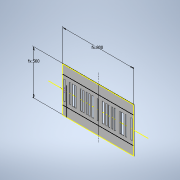
# Autodesk Inventor part: ferrite_layer_dex_1R1
Saved by Autodesk Inventor 2021 (Build 250183000, 183)
## iProperties
Created: 2021-01-27
Part Number: ferrite_layer_dex_1R1
Material: Generic
Document SubType Name: Modeling
Designer: pduy110
Density: 1 g/cm^3
Appearance: Default
Author: pduy110
Autodesk Inventor part; units mm, degrees
ref_plane "YZ Plane" through (0, 0, 0) normal (1, 0, 0) x (0, 1, 0)
ref_plane "XZ Plane" through (0, 0, 0) normal (0, 1, 0) x (-1, 0, 0)
ref_plane "XY Plane" through (0, 0, 0) normal (0, 0, 1) x (1, 0, 0)
sketch "ferrite_layer_outline_sketch" plane through (0, 0, 0) normal (0, 0, 1) x (1, 0, 0)
  line L0 (0, 250) -> (800, 250)
  line L1 (800, 250) -> (800, -250)
  line L2 (800, -250) -> (0, -250)
  line L3 (0, -250) -> (0, 250)
  line L4 (-160, 0) -> (960, 0) projected
  line L5 (400, 250) -> (400, -250) construction
  line L6 (400, 366.8869) -> (400, -324.3455) construction
  line L7 (400, 250) -> (400, -250)
  point P0 (0, 0)
  point P1 (0, 0)
  point P2 (0, 0)
  point P3 (0, 0)
  point P4 (20, 0)
  dimension "d0" = 800
  dimension "d1" = 500
  constraints: 14 end point, 3 coincident, 3 midpoint, 3 point on line, 2 parallel, 1 collinear, 1 horizontal, 1 perpendicular
  measures "d0" distance between parallel lines of L1 L3
  measures "d1" distance between parallel lines of L2 L0
extrude "Sheet Extrude" add sketch "ferrite_layer_outline_sketch" along normal blind 4
ref_plane "acrylic_sheet_plane" through (0, 0, 4) normal (0, 0, 1) x (1, 0, 0)
sketch "Sketch4" plane through (0, 0, 4) normal (0, 0, 1) x (1, 0, 0)
  line L0 (14.5, 109) -> (29.5, 109)
  line L1 (29.5, 109) -> (29.5, -109)
  line L2 (29.5, -109) -> (14.5, -109)
  line L3 (14.5, -109) -> (14.5, 109)
  line L4 (-12.6534, 0) -> (47.471, 0)
  line L5 (0, 250) -> (0, -250) projected
  line L6 (800, 250) -> (0, 250) projected
  line L7 (0, -250) -> (800, -250) projected
  point P0 (0, 0)
  point P1 (14.5, 0)
  point P2 (0, 0)
  dimension "d43" = 15
  dimension "d44" = 218
  dimension "d45" = 14.5
  constraints: 10 end point, 2 horizontal, 2 midpoint, 2 parallel, 2 point on line, 1 perpendicular
  measures "d43" distance between parallel lines of L1 L3
  measures "d44" distance between parallel lines of L2 L0
  measures "d45" distance between parallel lines of L5 L3
extrude "Extrusion9" cut sketch "Sketch4" against normal through all
pattern_linear "Rectangular Pattern 7 fer" count 7 spacing 126 along (1, 0, 0) of "Extrusion9"
pattern_linear "Rectangular Pattern 8 fer" count 8 spacing 108 along (1, 0, 0) of "Extrusion9"
pattern_linear "pattern_test_#_of_ferrites 9 fer" count 9 spacing 94.5 along (1, 0, 0) of "Extrusion9"
pattern_linear "Rectangular Pattern 10 fer" [suppressed]
pattern_linear "Rectangular Pattern 13" count 13 spacing 63 along (1, 0, 0) of "Extrusion9"
sketch "Sketch5" plane through (0, 0, 4) normal (0, 0, 1) x (1, 0, 0)
  line L0 (0, 250) -> (0, -250) projected
  line L1 (0, 150) -> (800, 150)
  line L2 (800, -250) -> (800, 250) projected
  line L3 (800, 250) -> (0, 250) projected
  line L4 (0, -250) -> (800, -250) projected
  line L5 (0, -150) -> (800, -150)
  point P0 (0, 0)
  dimension "d66" = 100
  dimension "d68" = 100
  constraints: 4 end point, 4 point on line, 1 horizontal, 1 perpendicular
  measures "d66" distance between parallel lines of L3 L1
  measures "d68" distance between parallel lines of L4 L5
sketch "Sketch11" plane through (0, 0, 4) normal (0, 0, 1) x (1, 0, 0)
  circle A0 centre (47, 57.75) radius 3
  line L0 (800, 250) -> (0, 250) projected
  line L1 (0, 250) -> (0, -250) projected
  circle A1 centre (47, -122) radius 3
  line L2 (0, -250) -> (800, -250) projected
  point P0 (0, 0)
  dimension "d85" = 6
  dimension "d86" = 192.25
  dimension "d87" = 47
  dimension "d88" = 6
  dimension "d89" = 128
  dimension "d90" = 47
  constraints: 2 centre point
  measures "d85" diameter of A0
  measures "d86" distance from line of L0 A0.centre
  measures "d87" distance from line of A0.centre L1
  measures "d88" diameter of A1
  measures "d89" distance from line of L2 A1.centre
  measures "d90" distance from line of L1 A1.centre
extrude "Extrusion15" cut sketch "Sketch11" against normal through all
sketch "Sketch12" plane through (0, 0, 4) normal (0, 0, 1) x (1, 0, 0)
  line L0 (0, -250) -> (800, -250) projected
  line L1 (43.5, 60.75) -> (50, 60.75)
  line L2 (50, 60.75) -> (50, -250)
  line L3 (50, -250) -> (43.5, -250)
  line L4 (43.5, -250) -> (43.5, 60.75)
  line L5 (0, 250) -> (0, -250) projected
  point P0 (0, 0)
  dimension "d97" = 310.75
  dimension "d98" = 6.5
  dimension "d99" = 43.5
  constraints: 8 end point, 2 parallel, 1 horizontal, 1 perpendicular, 1 point on line
  measures "d97" distance of L3.end L1.start
  measures "d98" distance between parallel lines of L4 L2
  measures "d99" distance between parallel lines of L5 L4
extrude "Extrusion17" cut sketch "Sketch12" against normal through all
equation "\"d0\" = track_length"
equation "\"d1\" = track_width"
equation "\"d43\" = ferrite_width"
equation "\"d44\" = ferrite_length"
equation "\"d45\" = gap_distance"
equation "\"d50\" = parameter_5"
equation "\"d62\" = test_parameter_5"
equation "\"track_length\" = 800"
equation "\"track_width\" = 500"
equation "\"gap_distance\" = 14.5"
equation "\"ferrite_length\" = 218"
equation "\"ferrite_width\" = 15"
equation "\"ferrite_height\" = 8"
equation "\"acrylic_sheet_8mm\" = 8"
equation "\"parameter_5\" = 126"
equation "\"test_parameter_5\" = 94.5"
body "Solid8"
